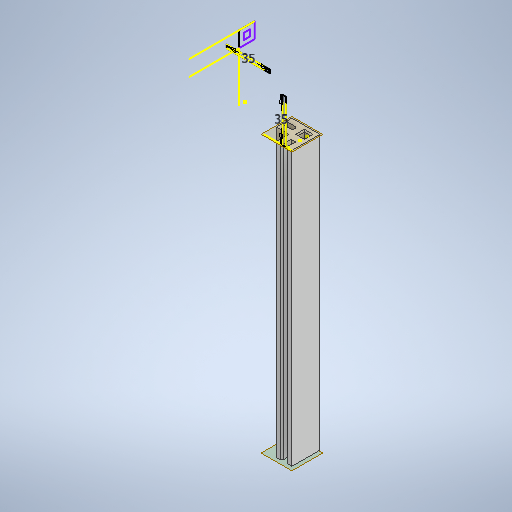
# Autodesk Inventor part: Kątownk 3mm_z_dziurą
Saved by Autodesk Inventor 2025 (Build 290162000, 162)
## iProperties
Created: 2025-07-29
Part Number: Kątownk 3mm_z_dziurą
Material: Ogólny
Document SubType Name: Modeling
Designer: ThePi
Density: 1 g/cm^3
Appearance: Domyślna
Author: ThePi
Autodesk Inventor part; units mm, degrees
ref_plane "YZ Plane" through (0, 0, 0) normal (1, 0, 0) x (0, 1, 0)
ref_plane "XZ Plane" through (0, 0, 0) normal (0, 1, 0) x (-1, 0, 0)
ref_plane "XY Plane" through (0, 0, 0) normal (0, 0, 1) x (1, 0, 0)
sketch "Szkic1" plane through (0, 0, 0) normal (0, 1, 0) x (-1, 0, 0)
  line L0 (0, 0) -> (0, 15)
  line L1 (0, 15) -> (0, 0)
  line L2 (0, 0) -> (15, 0)
  line L3 (3, 10) -> (4.25, 10)
  line L4 (3, 10) -> (1.75, 10)
  line L5 (1.75, 10) -> (1.75, 15)
  line L6 (4.25, 10) -> (4.25, 15)
  line L7 (1.75, 15) -> (-3.25, 15)
  line L8 (4.25, 15) -> (9.25, 15)
  line L9 (-3.25, 15) -> (-3.25, 0)
  line L10 (-3.25, 0) -> (15, 0)
  line L11 (-3.25, 0) -> (11.75, 0)
  line L12 (9.25, 15) -> (9.25, 5)
  line L13 (9.25, 5) -> (19.25, 5)
  line L14 (19.25, 5) -> (19.25, 0)
  line L15 (19.25, 0) -> (14.25, 0)
  line L16 (14.25, 0) -> (14.25, -2.5)
  line L17 (14.25, -2.5) -> (19.25, -2.5)
  line L18 (19.25, -2.5) -> (19.25, -7.5)
  line L19 (19.25, -7.5) -> (9.25, -7.5)
  line L20 (-3.25, 0) -> (-3.25, -7.5)
  line L21 (-3.25, -7.5) -> (9.25, -7.5)
  line L22 (3, 10) -> (3, -1.25)
  line L23 (3, -1.25) -> (14.25, -1.25)
  dimension "d0" = 15
  dimension "d6" = 1.25
  dimension "d7" = 1.25
  dimension "d9" = 5
  dimension "d10" = 5
  dimension "d13" = 10
  dimension "d14" = 10
  dimension "d15" = 5
  dimension "d16" = 5
  dimension "d17" = 2.5
  dimension "d18" = 5
  dimension "d19" = 10
  constraints: 48 end point, 7 perpendicular, 5 point on line, 4 vertical, 2 collinear, 2 horizontal, 1 midpoint, 1 parallel
  measures "d0" distance of L0.start L0.end
  measures "d6" distance of L3.start L3.end
  measures "d7" distance of L3.start L4.end
  measures "d9" distance of L5.end L7.end
  measures "d10" distance of L6.end L8.end
  measures "d13" distance of L8.end L12.end
  measures "d14" distance of L12.end L13.end
  measures "d15" distance of L13.end L14.end
  measures "d16" distance of L14.end L15.end
  measures "d17" distance of L15.end L16.end
  measures "d18" distance of L17.end L18.end
  measures "d19" distance of L18.end L19.end
extrude "Wyciągnięcie proste1" add sketch "Szkic1" along normal blind 30
sketch "Szkic2" plane through (0, 30, 0) normal (0, 1, 0) x (1, 0, 0)
  line L0 (3.25, 7.5) -> (-19.25, 7.5) projected
  line L1 (-19.25, -5) -> (-9.25, -5) projected
  line L2 (-19.25, 7.5) -> (-19.25, -5)
  line L3 (-19.25, -5) -> (-9.25, -5)
  line L4 (-9.25, -5) -> (-9.25, -15) projected
  line L5 (-9.25, -5) -> (-9.25, -15)
  line L6 (-1.75, -15) -> (3.25, -15) projected
  line L7 (-9.25, -15) -> (3.25, -15)
  line L8 (3.25, -15) -> (3.25, 7.5)
  line L9 (3.25, 7.5) -> (-19.25, 7.5)
  point P0 (0, 0)
  constraints: 12 end point, 3 perpendicular, 2 collinear, 1 vertical
extrude "Wyciągnięcie proste2" add sketch "Szkic2" along normal blind 30
sketch "Szkic3" plane through (0, 0, 0) normal (0, -1, 0) x (1, 0, 0)
  point P0 (0, 0)
sketch "Szkic4" plane through (-19.25, 0, -7.5) normal (-1, 0, 0) x (0, 0, 1)
  line L0 (0, 30) -> (12.5, 30)
  line L1 (12.5, 0) -> (12.5, 60) projected
  line L2 (12.5, 30) -> (12.5, 60)
  line L3 (12.5, 60) -> (0, 60)
  line L4 (0, 60) -> (0, 30)
  point P0 (7.5, 0)
  constraints: 8 end point, 2 perpendicular, 1 collinear, 1 midpoint
extrude "Wyciągnięcie proste3" add sketch "Szkic4" along normal blind 30
sketch "Szkic5" plane through (-9.25, 0, 5) normal (-1, 0, 0) x (0, 0, 1)
  line L0 (10, 0) -> (10, 60) projected
  line L1 (10, 30) -> (5, 30) projected
  line L2 (10, 60) -> (10, 30)
  line L3 (10, 30) -> (0, 30)
  line L4 (0, 30) -> (0, 60)
  line L5 (0, 60) -> (10, 60)
  point P0 (-5, 0)
  constraints: 8 end point, 2 perpendicular, 1 collinear, 1 vertical
extrude "Wyciągnięcie proste4" add sketch "Szkic5" along normal up to surface (40 mm away)
sketch "Szkic6" plane through (0, 30, 0) normal (0, -1, 0) x (1, 0, 0)
  line L0 (-14.25, 0) -> (-19.25, 0) projected
  line L1 (-14.25, 0) -> (-49.25, 0)
  line L2 (-49.25, -7.5) -> (-49.25, 15) projected
  line L3 (-49.25, 0) -> (-49.25, -2.5)
  line L4 (-49.25, -2.5) -> (-14.25, -2.5)
  line L5 (-14.25, -2.5) -> (-14.25, 0)
  line L6 (-14.25, 10) -> (-49.25, 10)
  line L7 (-4.25, 10) -> (-1.75, 10) projected
  point P0 (0, 0)
  constraints: 10 end point, 3 point on line, 2 perpendicular, 1 collinear, 1 horizontal, 1 vertical
extrude "Wyciągnięcie proste5" cut sketch "Szkic6" against normal blind 5
sketch "Szkic7" plane through (-1.75, 0, 15) normal (0, 0, 1) x (1, 0, 0)
  line L0 (-7.5, 30) -> (-17.5, 30) projected
  line L1 (-7.5, 30) -> (-17.5, 30)
  line L2 (-7.5, 30) -> (-7.5, 40)
  line L3 (5, 0) -> (5, 60) projected
  line L4 (-7.5, 30) -> (2.5, 30) construction
  line L5 (-7.5, 40) -> (-47.5, 40)
  line L6 (-47.5, 60) -> (-47.5, 30) projected
  line L7 (-47.5, 40) -> (-47.5, 30)
  line L8 (-47.5, 30) -> (-7.5, 30)
  point P0 (1.75, 0)
  dimension "d30" = 10
  dimension "d31" = 10
  dimension "d32" = 90
  constraints: 12 end point, 2 collinear, 2 perpendicular, 1 horizontal, 1 parallel, 1 point on line, 1 vertical
  measures "d30" distance of L0.start L0.end
  measures "d31" distance of L0.start L2.end
  measures "d32" angle of L4 L2
extrude "Wyciągnięcie proste6" cut sketch "Szkic7" against normal up to surface (10 mm away)
sketch "Szkic8" plane through (-49.25, 0, -7.5) normal (-1, 0, 0) x (0, 0, 1)
  point P0 (7.5, 0)
sketch "Szkic9" plane through (0, 0, 0) normal (0, -1, 0) x (1, 0, 0)
  point P0 (0, 0)
sketch "Szkic10" plane through (-49.25, 0, -7.5) normal (-1, 0, 0) x (0, 0, 1)
  line L0 (0, 0) -> (0, 60) projected
  line L1 (0, 30) -> (0, 52.5)
  line L2 (0, 52.5) -> (22.5, 52.5)
  line L3 (22.5, 0) -> (22.5, 60) projected
  line L4 (22.5, 52.5) -> (22.5, 40)
  line L5 (22.5, 40) -> (12.5, 40)
  line L6 (12.5, 40) -> (12.5, 30)
  line L7 (0, 30) -> (5, 30) projected
  line L8 (12.5, 30) -> (0, 30)
  line L9 (22.5, 52.5) -> (22.5, 60)
  line L10 (22.5, 60) -> (0, 60) projected
  line L11 (0, 60) -> (0, 52.5)
  line L12 (22.5, 52.5) -> (0, 52.5)
  point P0 (7.5, 0)
  dimension "d35" = 22.5
  dimension "d36" = 90
  dimension "d37" = 10
  constraints: 18 end point, 4 perpendicular, 3 collinear, 2 point on line, 1 midpoint
  measures "d35" distance of L1.start L1.end
  measures "d36" angle of L1 L2
  measures "d37" distance of L4.end L5.end
sketch "Szkic11" plane through (0, 0, 0) normal (0, -1, 0) x (1, 0, 0)
  point P0 (0, 0)
extrude "Wyciągnięcie proste7" cut sketch "Szkic10" against normal up to surface (52.5 mm away) contours L0 L10 L3 L2
sketch "Szkic12" plane through (-9.25, 0, 15) normal (0, 0, 1) x (1, 0, 0)
  line L0 (12.5, 52.5) -> (-40, 52.5) projected
  line L1 (12.5, 52.5) -> (-10, 52.5)
  line L2 (-10, 30) -> (-40, 30) projected
  line L3 (-10, 52.5) -> (-10, 30)
  line L4 (-10, 30) -> (12.5, 30)
  line L5 (12.5, 0) -> (12.5, 52.5) projected
  line L6 (12.5, 30) -> (12.5, 52.5)
  line L7 (-10, 30) -> (-10, 40)
  line L8 (-40, 40) -> (0, 40) projected
  line L9 (0, 40) -> (0, 30.3734)
  line L10 (0, 0) -> (0, 40) projected
  point P0 (9.25, 0)
  point P1 (0, 30)
  point P2 (0, 40)
  constraints: 12 end point, 3 perpendicular, 3 point on line, 1 parallel
extrude "Wyciągnięcie proste8" add sketch "Szkic12" against normal blind 10 contours L8 L9 L10 L4 L3
sketch "Szkic13" plane through (-9.25, 0, 15) normal (0, 0, 1) x (1, 0, 0)
  line L0 (-40, 52.5) -> (-40, 40) projected
  line L1 (-40, 40) -> (-40, 45)
  line L2 (-40, 45) -> (-10, 45)
  line L3 (-10, 45) -> (-10, 47.5)
  line L4 (-10, 47.5) -> (-40, 47.5)
  line L5 (12.5, 52.5) -> (-40, 52.5) projected
  line L6 (-40, 52.5) -> (-40, 47.5)
  line L7 (-40, 45) -> (-40, 47.5)
  point P0 (9.25, 0)
  dimension "d42" = 5
  dimension "d43" = 30
  dimension "d44" = 2.5
  constraints: 12 end point, 2 collinear, 2 perpendicular, 2 point on line, 1 horizontal
  measures "d42" distance of L0.end L1.end
  measures "d43" distance of L1.end L2.end
  measures "d44" distance of L2.end L3.end
extrude "Wyciągnięcie proste9" cut sketch "Szkic13" against normal blind 5
sketch "Szkic14" plane through (-9.25, 0, 15) normal (0, 0, 1) x (1, 0, 0)
  line L0 (12.5, 0) -> (12.5, 52.5) projected
  line L1 (12.5, 52.5) -> (-10, 52.5)
  line L2 (12.5, 52.5) -> (-40, 52.5) projected
  line L3 (-10, 40) -> (-10, 30) projected
  line L4 (-10, 52.5) -> (-10, 30)
  line L5 (-10, 30) -> (12.5, 30)
  line L6 (12.5, 30) -> (12.5, 52.5)
  point P0 (9.25, 0)
  constraints: 8 end point, 2 perpendicular, 1 point on line, 1 vertical
extrude "Wyciągnięcie proste10" add sketch "Szkic14" along normal blind 30
sketch "Szkic15" plane through (-1.75, 0, 15) normal (0, 0, 1) x (1, 0, 0)
  line L0 (0, 0) -> (0, 30) projected
  line L1 (0, 0) -> (0, 35)
  line L2 (0, 35) -> (0, 0)
  line L3 (-2.5, 0) -> (-2.5, 30) projected
  line L4 (0, 0) -> (-2.5, 0)
  line L5 (5, 0) -> (-17.5, 0) projected
  line L6 (-2.5, 0) -> (-2.5, 35)
  line L7 (-2.5, 35) -> (0, 35)
  line L8 (0, 0) -> (0, 35)
  line L9 (-17.5, 45) -> (-47.5, 45) projected
  line L10 (-47.5, 45) -> (-12.5, 45)
  line L11 (-12.5, 45) -> (-47.5, 45)
  line L12 (-47.5, 47.5) -> (-17.5, 47.5) projected
  line L13 (-47.5, 45) -> (-47.5, 47.5)
  line L14 (-47.5, 47.5) -> (-12.5, 47.5)
  line L15 (-12.5, 47.5) -> (-12.5, 45)
  point P0 (1.75, 0)
  point P1 (-17.5, 47.5)
  dimension "d49" = 35
  dimension "d50" = 35
  constraints: 22 end point, 6 collinear, 2 perpendicular, 2 vertical, 1 parallel
  measures "d49" distance of L0.start L1.end
  measures "d50" distance of L9.end L10.end
extrude "Wyciągnięcie proste11" cut sketch "Szkic15" against normal up to surface (5 mm away)
sketch "Szkic16" plane through (-9.25, 0, 45) normal (0, 0, 1) x (1, 0, 0)
  line L0 (7.5, 0) -> (7.5, 35) projected
  line L1 (7.5, 30) -> (7.5, 35)
  line L2 (5, 35) -> (5, 30) projected
  line L3 (7.5, 35) -> (5, 35)
  line L4 (5, 35) -> (5, 30)
  line L5 (5, 30) -> (7.5, 30)
  line L6 (-10, 40) -> (-10, 45) projected
  line L7 (-10, 45) -> (-5, 45) projected
  line L8 (-10, 45) -> (-5, 45)
  line L9 (-5, 47.5) -> (-10, 47.5) projected
  line L10 (-5, 45) -> (-5, 47.5)
  line L11 (-5, 47.5) -> (-10, 47.5)
  line L12 (-10, 47.5) -> (-10, 45)
  point P0 (9.25, 0)
  dimension "d53" = 5
  constraints: 16 end point, 5 perpendicular, 3 collinear, 1 point on line
  measures "d53" distance of L1.start L0.end
extrude "Wyciągnięcie proste12" cut sketch "Szkic16" against normal up to surface (35 mm away)
sketch "Szkic17" plane through (-9.25, 0, 45) normal (0, 0, 1) x (1, 0, 0)
  line L0 (-10, 30) -> (5, 30) projected
  line L1 (0, 30) -> (0, 40)
  line L2 (-40, 40) -> (-10, 40) projected
  line L3 (0, 40) -> (-10, 40)
  line L4 (-10, 40) -> (-10, 30)
  line L5 (-10, 30) -> (0, 30)
  point P0 (9.25, 0)
  dimension "d56" = 10
  constraints: 8 end point, 3 perpendicular, 1 point on line
  measures "d56" distance of L1.start L1.end
extrude "Wyciągnięcie proste13" cut sketch "Szkic17" against normal up to surface (40 mm away)
sketch "Szkic18" plane through (-49.25, 0, -7.5) normal (-1, 0, 0) x (0, 0, 1)
  line L0 (12.5, 0) -> (12.5, 40) projected
  line L1 (12.5, 40) -> (0, 40)
  line L2 (0, 52.5) -> (52.5, 52.5) projected
  line L3 (0, 40) -> (0, 52.5)
  line L4 (0, 52.5) -> (12.5, 52.5)
  line L5 (52.5, 40) -> (12.5, 40) projected
  line L6 (12.5, 40) -> (12.5, 52.5)
  line L7 (6.25, 43.75) -> (8.75, 43.75)
  line L8 (8.75, 43.75) -> (8.75, 48.75)
  line L9 (8.75, 48.75) -> (3.75, 48.75)
  line L10 (3.75, 48.75) -> (3.75, 43.75)
  line L11 (3.75, 43.75) -> (8.75, 43.75)
  point P0 (7.5, 0)
  constraints: 18 end point, 4 perpendicular, 2 point on line, 1 collinear
extrude "Wyciągnięcie proste14" cut sketch "Szkic18" against normal blind 17 contours L11 L10 L9 L8 L7
sketch "Szkic19" plane through (0, 0, 0) normal (0, -1, 0) x (1, 0, 0)
  line L0 (3.25, 15) -> (3.25, -7.5) projected
  line L1 (3.25, -7.5) -> (-19.25, -7.5) projected
  line L2 (-19.25, 5) -> (-9.25, 5) projected
  line L3 (-9.25, 5) -> (3.25, 5)
  line L4 (3.25, 5) -> (3.25, -7.5)
  line L5 (3.25, -7.5) -> (-9.25, -7.5)
  line L6 (-9.25, -7.5) -> (-9.25, 5)
  line L7 (-3, 1.25) -> (-5.5, 1.25)
  line L8 (-5.5, 1.25) -> (-5.5, -3.75)
  line L9 (-5.5, -3.75) -> (-0.5, -3.75)
  line L10 (-0.5, -3.75) -> (-0.5, 1.25)
  line L11 (-0.5, 1.25) -> (-5.5, 1.25)
  point P0 (0, 0)
  dimension "d65" = 2.5
  constraints: 18 end point, 5 perpendicular, 3 point on line
  measures "d65" distance of L7.start L7.end
extrude "Wyciągnięcie proste15" cut sketch "Szkic19" against normal blind 17 contours L11 L10 L9 L8 L7
sketch "Szkic20" plane through (-9.25, 0, 45) normal (0, 0, 1) x (1, 0, 0)
  line L0 (0, 0) -> (0, 40) projected
  line L1 (0, 40) -> (12.5, 40)
  line L2 (12.5, 0) -> (12.5, 52.5) projected
  line L3 (0, 40) -> (0, 52.5)
  line L4 (-40, 52.5) -> (12.5, 52.5) projected
  line L5 (0, 52.5) -> (12.5, 52.5)
  line L6 (12.5, 52.5) -> (12.5, 40)
  line L7 (8.75, 46.25) -> (8.75, 43.75)
  line L8 (8.75, 43.75) -> (3.75, 43.75)
  line L9 (3.75, 43.75) -> (3.75, 48.75)
  line L10 (3.75, 48.75) -> (8.75, 48.75)
  line L11 (8.75, 48.75) -> (8.75, 43.75)
  point P0 (9.25, 0)
  constraints: 18 end point, 3 perpendicular, 3 point on line, 2 collinear, 1 horizontal, 1 vertical
extrude "Wyciągnięcie proste16" cut sketch "Szkic20" against normal blind 17 contours L7 L8 L9 L10 L11
chamfer "Faza1" distance 1 angle 45 12 edges at (-3, 0, 1.25) (-5.5, 0, -1.25) (-0.5, 0, -1.25) (-3, 0, -3.75) (-0.5, 46.25, 45) (-3, 48.75, 45) (-5.5, 46.25, 45) (-3, 43.75, 45) (-49.25, 48.75, -1.25) (-49.25, 46.25, -3.75) (-49.25, 43.75, -1.25) (-49.25, 46.25, 1.25)
thicken "Pogrubienie2" operation cut thickness 0.5 both sides no extend neighbours no toward (0, 1, 0) faces at (-27.5833, 47.5, 11.6667)
thicken "Pogrubienie4" operation cut thickness 0.5 both sides no extend neighbours no toward (0, -1, 0) faces at (-27.5833, 45, 11.6667)
thicken "Pogrubienie5" operation cut thickness 0.5 both sides no extend neighbours no toward (0, 0, -1) faces at (-15.9167, 21.6667, -2.5)
thicken "Pogrubienie6" operation cut thickness 0.5 both sides no extend neighbours no toward (0, 0, 1) faces at (-27.5833, 33.3333, 0)
thicken "Pogrubienie8" operation cut thickness 2.5 both sides no extend neighbours no toward (0, 0, -1) faces at (-2.5833, 23.3333, 10) (-2.5833, 35, 33.3333)
thicken "Pogrubienie9" operation cut thickness 2.5 both sides no extend neighbours no toward (0, 1, 0) faces at (-25.9167, 35, -0.6667) (-14.25, 11.6667, -0.6667)
thicken "Pogrubienie10" operation cut thickness 2.5 both sides no extend neighbours no toward (1, 0, 0) faces at (-14.25, 45.6667, 33.3333) (-25.9167, 46.8333, 10)
sketch "Szkic21" plane through (-19.25, 0, 5) normal (0, 0, 1) x (1, 0, 0)
  point P0 (19.25, 0)
sketch "Szkic22" plane through (0, 0, 0) normal (0, -1, 0) x (1, 0, 0)
  arc A0 (-11.75, -3) -> (-11.75, 0.5) centre (-12.7182, -1.25) ccw
  line L0 (-11.75, 0.5) -> (-11.75, -3) projected
  line L1 (-11.75, -3) -> (-11.75, 0.5)
  point P0 (0, 0)
  dimension "d100" = 2
  constraints: 2 end point, 2 point on circle, 1 centre point, 1 collinear
  measures "d100" radius of A0
extrude "Wyciągnięcie proste17" cut sketch "Szkic22" against normal up to surface (37.5 mm away)
sketch "Szkic23" plane through (-19.25, 0, 5) normal (0, 0, 1) x (1, 0, 0)
  line L0 (7.5, 0) -> (7.5, 37.5) projected
  line L1 (7.5, 0) -> (7.5, 37.5)
  line L2 (7.5, 37.5) -> (-30, 37.5) projected
  line L3 (7.5, 37.5) -> (9, 37.5)
  line L4 (9, 37.5) -> (9, 34.5)
  line L5 (9, 34.5) -> (6, 34.5)
  line L6 (6, 34.5) -> (6, 37.5)
  line L7 (6, 37.5) -> (9, 37.5)
  line L8 (9, 37.5) -> (8.3928, 37.5)
  line L9 (8.3928, 37.5) -> (8.3928, 34.5)
  point P0 (19.25, 0)
  point P1 (6, 37.5)
  point P2 (8.3928, 37.5)
  dimension "d103" = 3
  dimension "d104" = 3
  constraints: 16 end point, 5 perpendicular, 3 point on line, 1 collinear, 1 vertical
  measures "d103" distance of L3.end L4.end
  measures "d104" distance of L4.end L5.end
extrude "Wyciągnięcie proste18" cut sketch "Szkic23" against normal blind 5.5 contours L5 L6 L2 L0 | L0 L3 L9 L5
chamfer "Faza4" distance 1 angle 45 4 edges at (-10.8572, 36, 5) (-12.0536, 34.5, 5) (-13.25, 36, 5) (-12.0536, 37.5, 5)
thicken "Pogrubienie11" operation cut thickness 0.5 both sides no extend neighbours no toward (-1, 0, 0) faces at (-4.25, 35, 22.5)
thicken "Pogrubienie12" operation cut thickness 0.5 both sides no extend neighbours no toward (1, 0, 0) faces at (-1.75, 22.5, 10)
chamfer "Faza5" distance 1 angle 45 12 edges at (-4.75, 15, 15) (-4.75, 30, 30) (-1.25, 30, 30) (-1.25, 15, 15) (-19.25, 15, 0.5) (-34.25, 30, 0.5) (-34.25, 30, -3) (-19.25, 15, -3) (-34.25, 48, 15) (-34.25, 44.5, 15) (-19.25, 44.5, 30) (-19.25, 48, 30)
sketch "Szkic24" plane through (0, 0, 0) normal (0, -1, 0) x (1, 0, 0)
  line L0 (-19.25, -4) -> (-18.25, -3) projected
  line L1 (-19.25, -7.5) -> (-19.25, -4) projected
  line L2 (3.25, -7.5) -> (-19.25, -7.5) projected
  line L3 (3.25, 15) -> (3.25, -7.5) projected
  line L4 (-0.25, 15) -> (3.25, 15) projected
  line L5 (-1.25, 14) -> (-0.25, 15) projected
  line L6 (-1.25, 14) -> (-1.25, 7.5) projected
  line L7 (-1.25, 7.5) -> (-4.75, 7.5) projected
  line L8 (-4.75, 7.5) -> (-4.75, 14) projected
  line L9 (-5.75, 15) -> (-4.75, 14) projected
  line L10 (-9.25, 15) -> (-5.75, 15) projected
  line L11 (-9.25, 5) -> (-9.25, 15) projected
  line L12 (-19.25, 5) -> (-9.25, 5) projected
  line L13 (-19.25, 1.5) -> (-19.25, 5) projected
  line L14 (-18.25, 0.5) -> (-19.25, 1.5) projected
  line L15 (-18.25, 0.5) -> (-11.75, 0.5) projected
  arc A0 (-11.75, -3) -> (-11.75, 0.5) centre (-12.7182, -1.25) ccw projected
  line L16 (-11.75, -3) -> (-18.25, -3) projected
  line L17 (-6.5, -4.75) -> (0.5, -4.75) projected
  line L18 (-6.5, 2.25) -> (-6.5, -4.75) projected
  line L19 (0.5, 2.25) -> (-6.5, 2.25) projected
  line L20 (0.5, -4.75) -> (0.5, 2.25) projected
  line L21 (-5.5, -3.75) -> (-5.5, 1.25) projected
  line L22 (-0.5, 1.25) -> (-0.5, -3.75) projected
  line L23 (-5.5, 1.25) -> (-0.5, 1.25) projected
  line L24 (-0.5, -3.75) -> (-5.5, -3.75) projected
  line L25 (0.5, 2.25) -> (-6.5, 2.25) projected
  line L26 (-6.5, 2.25) -> (-6.5, -4.75) projected
  line L27 (-5.5, -3.75) -> (-5.5, 1.25) projected
  line L28 (-5.5, 1.25) -> (-0.5, 1.25) projected
  line L29 (-0.5, 1.25) -> (-0.5, -3.75) projected
  line L30 (-0.5, -3.75) -> (-5.5, -3.75) projected
  point P0 (0, 0)
extrude "Wyciągnięcie proste19" add sketch "Szkic24" along normal blind 220 separate body contours L0 L16 A0 L15 L14 L13 L12 L11 L10 L9 L8 L7 L6 L5 L4 L3 L2 L1 | L18 L19 L20 L17 | L21 L23 L22 L24
ref_plane "Płaszczyzna konstrukcyjna1" through (0, -222, 0) normal (0, -1, 0) x (1, 0, 0)
sketch "Szkic26" plane through (0, -222, 0) normal (0, -1, 0) x (1, 0, 0)
  line L0 (-5.5, -3.75) -> (-5.5, 1.25) projected
  line L1 (-5.5, 1.25) -> (-0.5, 1.25) projected
  line L2 (-0.5, 1.25) -> (-0.5, -3.75) projected
  line L3 (-0.5, -3.75) -> (-5.5, -3.75) projected
  point P0 (0, 0)
extrude "Wyciągnięcie proste20" cut sketch "Szkic26" against normal blind 17
chamfer "Faza6" distance 1 angle 45 4 edges at (-5.5, -220, -1.25) (-3, -220, -3.75) (-0.5, -220, -1.25) (-3, -220, 1.25)
ref_plane "Płaszczyzna konstrukcyjna2" through (0, 0, 0) normal (0, 1, 0) x (1, 0, 0)
sketch "Szkic27" plane through (0, 0, 0) normal (0, 1, 0) x (1, 0, 0)
  line L0 (-5.5, 3.75) -> (-5.5, -1.25) projected
  line L1 (-5.5, -1.25) -> (-0.5, -1.25) projected
  line L2 (-0.5, -1.25) -> (-0.5, 3.75) projected
  line L3 (-0.5, 3.75) -> (-5.5, 3.75) projected
  point P0 (0, 0)
extrude "Wyciągnięcie proste21" cut sketch "Szkic27" against normal blind 17
chamfer "Faza7" distance 1 angle 45 4 edges at (-5.5, 0, -1.25) (-3, 0, 1.25) (-3, 0, -3.75) (-0.5, 0, -1.25)
